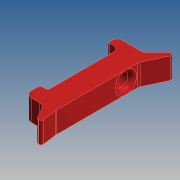
# Autodesk Inventor part: P104
Saved by Autodesk Inventor 2019 (Build 230136000, 136)
## iProperties
Created: 2016-10-17
Part Number: P104
Material: ABS Plastic
Document SubType Name: Modeling
Designer: serge.amoos
Density: 1.06 g/cm^3
Appearance: Light Red
Description: Levier 1
Author: serge.amoos
Autodesk Inventor part; units mm, degrees
ref_plane "YZ Plane" through (0, 0, 0) normal (1, 0, 0) x (0, 1, 0)
ref_plane "XZ Plane" through (0, 0, 0) normal (0, 1, 0) x (-1, 0, 0)
ref_plane "XY Plane" through (0, 0, 0) normal (0, 0, 1) x (1, 0, 0)
sketch "Sketch1" plane through (0, 0, 0) normal (0, 0, 1) x (1, 0, 0)
  line L0 (20, -22) -> (4.1, -22) construction
  line L1 (4.1, -22) -> (4.1, -25) construction
  line L2 (4.1, -25) -> (0, -25) construction
  line L3 (30, -47) -> (20, -47) construction
  circle A0 centre (17, -17) radius 3 construction
  line L4 (14, -17) -> (14, 0) construction
  line L5 (14, 0) -> (30, 0) construction
  line L6 (20, -47) -> (20, -17) construction
  line L7 (20, -47) -> (30, -47) construction
  line L8 (30, -47) -> (30, 0) construction
  line L9 (0, -25) -> (0, 0) construction
  line L10 (30, 0) -> (30, -47) construction
  line L11 (-7.0263, 0) -> (42.1581, 0) construction
  line L12 (0, -63.6142) -> (0, 17.6853) construction
  line L13 (17, -17) -> (17, -8) construction
  circle A1 centre (17, -8) radius 3 construction
  line L14 (16.5, -38) -> (20, -38)
  line L15 (16.5, -45) -> (25, -45)
  line L16 (25, -45) -> (29.0415, -52)
  line L17 (29.0415, -52) -> (31, -52)
  line L18 (31, -52) -> (30, -44.4042)
  line L19 (30, -44.4042) -> (30, -1)
  line L20 (15, -1) -> (30, -1)
  line L21 (15, -1) -> (15, -5.7639)
  line L22 (16.5, -45) -> (16.5, -38)
  arc A2 (20, -8) -> (15, -5.7639) centre (17, -8) ccw
  line L23 (20, -8) -> (20, -38)
  line L24 (27, -1) -> (34.0711, 6.0711)
  line L25 (34.0711, 6.0711) -> (35.1317, 5.0104)
  line L26 (30, -6) -> (35.1317, 5.0104)
  point P0 (0, 0)
  point P1 (0, 0)
  dimension "d10" = 6
  dimension "d1" = 3
  dimension "d2" = 5
  dimension "d3" = 14
  dimension "d4" = 20
  dimension "d5" = 22
  dimension "d6" = 30
  dimension "d7" = 4.1
  dimension "d8" = 3
  dimension "d9" = 25
  dimension "d11" = 9
  dimension "d12" = 0
  dimension "d13" = 16
  dimension "d14" = 7
  dimension "d15" = 3.5
  dimension "d16" = 120
  dimension "d17" = 7.5
  dimension "d19" = 5
  dimension "d20" = 5
  dimension "d21" = 1
  dimension "d22" = 1
  dimension "d23" = 1
  dimension "d40" = 45
  dimension "d41" = 3
  dimension "d42" = 10
  dimension "d43" = 5
  dimension "d46" = 1.5
  constraints: 50 end point, 4 collinear, 4 perpendicular, 4 point on circle, 4 point on line, 4 vertical, 3 coincident, 2 centre point, 1 horizontal, 1 parallel, 1 tangent, 4 other
  measures "d1" radius of A0
  measures "d2" distance from line of L0 L13.start
  measures "d3" distance between parallel lines of L4 L12
  measures "d4" distance between parallel lines of L6 L12
  measures "d5" distance between parallel lines of L0 L11
  measures "d6" distance between parallel lines of L12 L8
  measures "d7" distance between parallel lines of L12 L1
  measures "d8" distance between parallel lines of L0 L2
  measures "d9" distance between parallel lines of L7 L0
  measures "d11" distance of L13.start L13.end
  measures "d12" angle of L4 L13
  measures "d13" distance between parallel lines of L14 L0
  measures "d14" distance of L15.start L14.start
  measures "d15" distance between parallel lines of L6 L22
  measures "d16" angle of L16 L15
  measures "d17" angle of L19 L18
  measures "d19" distance between parallel lines of L17 L7
  measures "d20" distance from line of L15.end L6
  measures "d21" distance from line of L19 L17.end
  measures "d22" distance between parallel lines of L20 L11
  measures "d23" distance between parallel lines of L4 L21
  measures "d40" angle of L24 L20
  measures "d41" distance from line of L8 L24.start
  measures "d42" distance from line of L24.start L25
  measures "d43" distance of L26.start L19.end
  measures "d46" distance of L24.end L25.end
extrude "Extrusion1" add sketch "Sketch1" along normal mid plane 9.8
fillet "Fillet1" radius 0.5 1 edges at (15, -5.7639, 0)
fillet "Fillet2" radius 1 2 edges at (29.0415, -52, 0) (31, -52, 0)
fillet "Fillet3" radius 3 3 edges at (16.5, -45, 0) (25, -45, 0) (30, -44.4042, 0)
fillet "Fillet4" radius 2 1 edges at (15, -1, 0)
fillet "Fillet5" radius 1 1 edges at (20, -38, 0)
sketch "Sketch2" plane through (30, -44.2076, 4.9) normal (1, 0, 0) x (0, 0, -1)
  line L0 (-1.96, 44.2076) -> (11.76, 44.2076) construction
  line L1 (4.9, -19.4066) -> (4.9, 61.8929) construction
  point P0 (4.9, 44.2076)
  point P1 (4.9, 32.2076)
  dimension "d44" = 12
  constraints: 1 point on line
  measures "d44" distance from line of point (4.9, 32.208) L0
hole "Hole1" at (30, -12, 0) direction (-1, 0, 0) diameter 6 end through all
fillet "Fillet6" radius 2 2 edges at (30, -12, 3) (20, -12, 3)
fillet "Fillet8" radius 1 2 edges at (34.0711, 6.0711, 0) (35.1317, 5.0104, 0)
fillet "Fillet9" radius 2 1 edges at (27, -1, 0)
fillet "Fillet10" radius 1 1 edges at (16.5, -38, 0)
fillet "Fillet11" radius 2 1 edges at (30, -6, 0)
body "Solid1"
